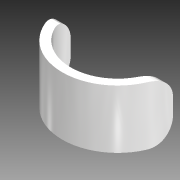
# Autodesk Inventor part: FE-120-004 Pivot Hardstop
Saved by Autodesk Inventor 2021 (Build 250183000, 183)
## iProperties
Created: 2021-01-11
Part Number: FE-120-004 Pivot Hardstop
Material: PVC-Piping
Document SubType Name: Modeling
Density: 1.4 g/cm^3
Appearance: Smooth - White
Autodesk Inventor part; units mm, degrees
ref_plane "YZ Plane" through (0, 0, 0) normal (1, 0, 0) x (0, 1, 0)
ref_plane "XZ Plane" through (0, 0, 0) normal (0, 1, 0) x (-1, 0, 0)
ref_plane "XY Plane" through (0, 0, 0) normal (0, 0, 1) x (1, 0, 0)
sketch "Sketch1" plane through (0, 0, 0) normal (0, 1, 0) x (-1, 0, 0)
  arc A0 (24.13, 0) -> (-24.13, 0) centre (0, 0) ccw
  arc A1 (20.447, 0) -> (-20.447, 0) centre (0, 0) ccw
  line L0 (24.13, 0) -> (-24.13, 0)
  dimension "d0" = 48.26
  dimension "d1" = 40.894
  constraints: 4 point on circle, 2 centre point, 2 coincident, 2 end point, 2 point on line, 1 horizontal, 1 midpoint
  measures "d0" diameter of A0
  measures "d1" diameter of A1
extrude "Extrusion1" add sketch "Sketch1" along normal mid plane 25.4 contours L0 A1 A0
fillet "Fillet1" radius 9.525 4 edges at (-22.2885, 12.7, 0) (-22.2885, -12.7, 0) (22.2885, -12.7, 0) (22.2885, 12.7, 0)
body "Solid1"
